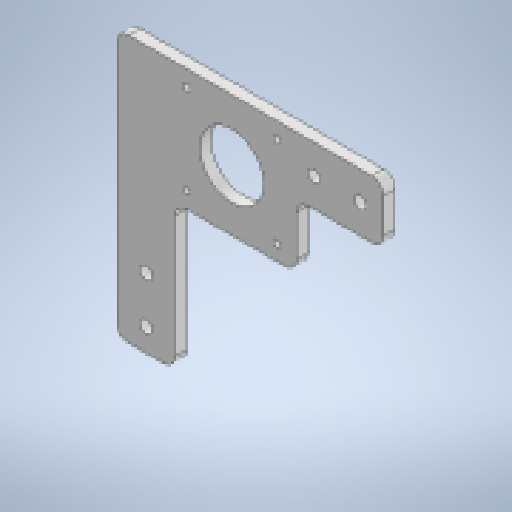
# Autodesk Inventor part: креп_мотора
Saved by Autodesk Inventor 2023.1 (Build 271208000, 208)
## iProperties
Created: 2025-11-24
Part Number: креп_мотора
Material: Типовые
Document SubType Name: Modeling
Designer: DELL
Density: 1 g/cm^3
Appearance: По умолчанию
Author: DELL
Autodesk Inventor part; units mm, degrees
ref_plane "YZ Plane" through (0, 0, 0) normal (1, 0, 0) x (0, 1, 0)
ref_plane "XZ Plane" through (0, 0, 0) normal (0, 1, 0) x (-1, 0, 0)
ref_plane "XY Plane" through (0, 0, 0) normal (0, 0, 1) x (1, 0, 0)
sketch "Эскиз1" plane through (0, 0, 0) normal (0, 0, 1) x (1, 0, 0)
  line L0 (-34.95, 71) -> (-39.5, 71) projected
  line L1 (-39.5, 71) -> (52.5, 71)
  line L2 (52.5, 71) -> (52.5, 51)
  line L3 (-19.5, -21) -> (-39.5, -21)
  line L4 (-39.5, -21) -> (-39.5, 71)
  line L5 (-21, 66.8757) -> (-21, 32.8243) construction
  line L6 (-19.5, 71) -> (22.5, 71)
  line L7 (22.5, 51) -> (22.5, 29)
  line L8 (22.5, 29) -> (-19.5, 29)
  line L9 (-19.5, 29) -> (-19.5, 71)
  line L10 (-19.5, 29) -> (22.5, 29)
  line L11 (-19.5, -21) -> (-19.5, 29)
  line L12 (22.5, 29) -> (22.5, 51)
  line L13 (22.5, 51) -> (52.5, 51)
  dimension "d14" = 92
  dimension "d20" = 20
  dimension "d21" = 42
  dimension "d22" = 42
  dimension "d24" = 92
  dimension "d25" = 30
  constraints: 24 end point, 4 parallel, 4 perpendicular, 3 horizontal, 1 point on line
  measures "d14" distance of L3.end L0.end
  measures "d20" distance of L1.end L2.end
  measures "d21" distance of L6.end L7.end
  measures "d22" distance of L7.end L8.end
  measures "d24" distance of L0.end L1.end
  measures "d25" distance of L7.start L2.end
extrude "Выдавливание1" add sketch "Эскиз1" along normal blind 4
sketch "Эскиз2" plane through (0, 0, 4) normal (0, 0, 1) x (1, 0, 0)
  circle A0 centre (0.15, 49.85) radius 11 projected
  line L0 (52.5, 51) -> (52.5, 71) projected
  line L1 (52.5, 61) -> (-39.5, 61) construction
  line L2 (-39.5, 71) -> (-39.5, -21) projected
  line L3 (-39.5, -21) -> (-19.5, -21) projected
  line L4 (-29.5, -21) -> (-29.5, 71) construction
  line L5 (52.5, 71) -> (-39.5, 71) projected
  circle A1 centre (44.5, 61) radius 2.1
  circle A2 centre (28.5, 61) radius 2.1
  circle A3 centre (-15.35, 34.35) radius 1.25 projected
  circle A4 centre (15.65, 34.35) radius 1.25 projected
  circle A5 centre (15.65, 65.35) radius 1.25 projected
  circle A6 centre (-15.35, 65.35) radius 1.25 projected
  line L6 (-39.5, 71) -> (-29.5, 61) construction
  circle A7 centre (-29.5, -13) radius 2.1
  circle A8 centre (-29.5, 3) radius 2.1
  dimension "d26" = 4.2
  dimension "d27" = 4.2
  dimension "d28" = 8
  dimension "d29" = 16
  constraints: 6 end point, 6 point on line, 4 centre point, 2 midpoint, 2 symmetric about line, 1 horizontal, 1 vertical, 2 other
  measures "d26" diameter of A1
  measures "d27" diameter of A2
  measures "d28" distance from line of A1.centre L0
  measures "d29" distance of A1.centre A2.centre
extrude "Выдавливание2" cut sketch "Эскиз2" against normal blind 4
fillet "Сопряжение1" radius 4 8 edges at (-39.5, -21, 2) (-19.5, -21, 2) (-19.5, 29, 2) (22.5, 29, 2) (22.5, 51, 2) (52.5, 51, 2) (52.5, 71, 2) (-39.5, 71, 2)
